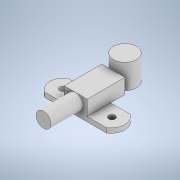
# Autodesk Inventor part: Latch
Saved by Autodesk Inventor 2020 (Build 240168000, 168)
## iProperties
Created: 2022-03-21
Part Number: Latch
Material: Genérico
Document SubType Name: Modeling
Designer: aarco
Density: 1 g/cm^3
Appearance: Valor por defecto
Author: aarco
Autodesk Inventor part; units mm, degrees
ref_plane "YZ Plane" through (0, 0, 0) normal (1, 0, 0) x (0, 1, 0)
ref_plane "XZ Plane" through (0, 0, 0) normal (0, 1, 0) x (-1, 0, 0)
ref_plane "XY Plane" through (0, 0, 0) normal (0, 0, 1) x (1, 0, 0)
sketch "Boceto1" plane through (0, 0, 0) normal (0, 1, 0) x (-1, 0, 0)
  line L0 (11.5, 5.5) -> (-11.5, 5.5)
  line L1 (-11.5, 5.5) -> (-11.5, -5.5)
  line L2 (-11.5, -5.5) -> (11.5, -5.5)
  line L3 (11.5, -5.5) -> (11.5, 5.5)
  line L4 (0, 0) -> (0, -30.7966)
  line L5 (0, 0) -> (-20.4633, 0)
  circle A0 centre (11.5, 0) radius 1.5
  circle A1 centre (-11.5, 0) radius 1.5
  line L6 (11.5, 5.5) -> (17.5, 5.5)
  line L7 (17.5, 5.5) -> (17.5, -5.5)
  line L8 (17.5, -5.5) -> (11.5, -5.5)
  line L9 (-11.5, -5.5) -> (-17.5, -5.5)
  line L10 (-17.5, -5.5) -> (-17.5, 5.5)
  line L11 (-17.5, 5.5) -> (-11.5, 5.5)
  arc A2 (14.5, -5.5) -> (14.5, 5.5) centre (10.9583, 0) ccw
  arc A3 (-14.5, 5.5) -> (-14.5, -5.5) centre (-10.9583, 0) ccw
  point P0 (0, -5.5)
  dimension "d0" = 23
  dimension "d1" = 11
  dimension "d2" = 3
  dimension "d3" = 3
  dimension "d4" = 35
  constraints: 24 end point, 7 midpoint, 5 perpendicular, 4 centre point, 4 point on circle, 4 point on line, 3 horizontal, 2 parallel, 2 tangent, 1 coincident, 1 symmetric about line, 1 vertical
  measures "d0" distance of L0.start L0.end
  measures "d1" distance of L2.end L0.start
  measures "d2" diameter of A0
  measures "d3" diameter of A1
  measures "d4" distance between parallel lines of L10 L7
extrude "Extrusión1" add sketch "Boceto1" along normal blind 2.2 contours L3 A0 L2 L4 L5 A1 L1 L0 | L6 A2 L8 L3 A0 | L1 A1 L5 A3 L11 | L5 L4 L2 L1 A1 | A1 L1 L9 A3 L5
sketch "Boceto2" plane through (0, 2.2, 0) normal (0, 1, 0) x (1, 0, 0)
  line L0 (-5.3885, 12.2229) -> (5.3885, 12.2229)
  line L1 (5.3885, 12.2229) -> (5.3885, -5.5)
  line L2 (5.3885, -5.5) -> (-5.3885, -5.5)
  line L3 (-5.3885, -5.5) -> (-5.3885, 12.2229)
  line L4 (-14.5, -5.5) -> (14.5, -5.5) projected
  line L5 (-3.5, -5.5) -> (3.5, -5.5)
  line L6 (3.5, -5.5) -> (3.5, -20.5)
  line L7 (3.5, -20.5) -> (-3.5, -20.5)
  line L8 (-3.5, -20.5) -> (-3.5, -5.5)
  circle A0 centre (0, 17.6115) radius 5.3885
  line L9 (-5.3885, 12.2229) -> (-5.3885, 43.935) construction
  line L10 (5.3885, 12.2229) -> (5.3885, 43.935) construction
  line L11 (0, 23) -> (-9.6882, 23)
  point P0 (0, 0)
  point P1 (0, -5.5)
  point P2 (0, -5.5)
  point P3 (0, 12.2229)
  dimension "d7" = 7
  dimension "d8" = 20.5
  dimension "d9" = 43.5
  constraints: 22 end point, 5 horizontal, 4 midpoint, 4 parallel, 4 vertical, 2 perpendicular, 3 other
  measures "d7" distance of L6.end L7.end
  measures "d8" distance from line of point (0, 0) L7
  measures "d9" distance between parallel lines of L7 L11
extrude "Extrusión2" add sketch "Boceto2" along normal blind 7
fillet "Empalme1" radius 3.5 4 edges at (3.5, 9.2, 13) (-3.5, 9.2, 13) (3.5, 2.2, 13) (-3.5, 2.2, 13)
sketch "Boceto3" plane through (0, 9.2, -17.6115) normal (0, 1, 0) x (1, 0, 0)
  circle A0 centre (0, 0) radius 5.3885 projected
  point P0 (0, -17.6115)
  point P1 (0, -5.3885)
  constraints: 1 vertical alignment
extrude "Extrusión3" add sketch "Boceto3" along normal blind 4.5
